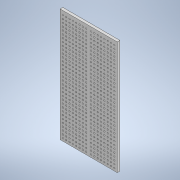
# Autodesk Inventor part: PCB_BOARD
Saved by Autodesk Inventor 2020 (Build 240168000, 168)
## iProperties
Created: 2020-06-08
Part Number: PCB_BOARD
Material: Generic
Document SubType Name: Modeling
Designer: Gebruiker
Density: 1 g/cm^3
Appearance: Default
Author: Gebruiker
Autodesk Inventor part; units mm, degrees
(part 1 of 2)
ref_plane "YZ Plane" through (0, 0, 0) normal (1, 0, 0) x (0, 1, 0)
ref_plane "XZ Plane" through (0, 0, 0) normal (0, 1, 0) x (-1, 0, 0)
ref_plane "XY Plane" through (0, 0, 0) normal (0, 0, 1) x (1, 0, 0)
sketch "Sketch1" plane through (0, 0, 0) normal (0, 0, 1) x (1, 0, 0)
  line L0 (-21.5, 42.5) -> (21.5, 42.5)
  line L1 (21.5, 42.5) -> (21.5, -42.5)
  line L2 (21.5, -42.5) -> (-21.5, -42.5)
  line L3 (-21.5, -42.5) -> (-21.5, 42.5)
  line L4 (-21.5, 32) -> (21.5, 32) construction
  line L5 (-21.7358, 34.5) -> (21.2642, 34.5) construction
  line L6 (-21.5945, 37) -> (21.4055, 37) construction
  line L7 (-33.8203, 0) -> (28.8511, 0) construction
  line L8 (-20.9841, 29.5) -> (22.0159, 29.5) construction
  line L9 (-20.1778, 24.5) -> (22.8222, 24.5) construction
  line L10 (-20.9207, 17) -> (22.0793, 17) construction
  line L11 (-20.9858, 19.5) -> (22.0142, 19.5) construction
  line L12 (-20.8573, 22) -> (22.1427, 22) construction
  line L13 (-21.1161, 27) -> (21.8839, 27) construction
  circle A0 centre (-19.3202, 39.5) radius 0.5
  circle A1 centre (-16.8202, 39.5) radius 0.5
  circle A2 centre (-14.3202, 39.5258) radius 0.5
  circle A3 centre (-11.8202, 39.5258) radius 0.5
  circle A4 centre (-9.3202, 39.5259) radius 0.5
  circle A5 centre (-6.8202, 39.5259) radius 0.5
  circle A6 centre (-4.3202, 39.5261) radius 0.5
  circle A7 centre (-1.8202, 39.5261) radius 0.5
  line L14 (0, 43.3712) -> (0, -59.117)
  circle A8 centre (19.3202, 39.5) radius 0.5
  circle A9 centre (16.8202, 39.5) radius 0.5
  circle A10 centre (14.3202, 39.5258) radius 0.5
  circle A11 centre (11.8202, 39.5258) radius 0.5
  circle A12 centre (9.3202, 39.5259) radius 0.5
  circle A13 centre (6.8202, 39.5259) radius 0.5
  circle A14 centre (1.8202, 39.5261) radius 0.5
  circle A15 centre (4.3202, 39.5261) radius 0.5
  line L15 (-21.5, 38.2501) -> (21.5, 38.2501) construction
  circle A16 centre (-19.3202, 37.0001) radius 0.5
  circle A17 centre (-16.8202, 37.0001) radius 0.5
  circle A18 centre (-14.3202, 36.9744) radius 0.5
  circle A19 centre (-11.8202, 36.9744) radius 0.5
  circle A20 centre (-9.3202, 36.9742) radius 0.5
  circle A21 centre (-6.8202, 36.9742) radius 0.5
  circle A22 centre (-1.8202, 36.9741) radius 0.5
  circle A23 centre (-4.3202, 36.9741) radius 0.5
  line L16 (0, 33.1289) -> (0, 135.6171)
  circle A24 centre (1.8202, 36.9741) radius 0.5
  circle A25 centre (4.3202, 36.9741) radius 0.5
  circle A26 centre (6.8202, 36.9742) radius 0.5
  circle A27 centre (9.3202, 36.9742) radius 0.5
  circle A28 centre (11.8202, 36.9744) radius 0.5
  circle A29 centre (14.3202, 36.9744) radius 0.5
  circle A30 centre (16.8202, 37.0001) radius 0.5
  circle A31 centre (19.3202, 37.0001) radius 0.5
  line L17 (-21.5945, 37) -> (0, 34.5) construction
  line L18 (0, 37) -> (-21.5, 34.5) construction
  line L19 (-21.5, 35.75) -> (21.5, 35.75) construction
  line L20 (-21.5945, 34.5) -> (21.4055, 34.5) construction
  circle A32 centre (-19.3202, 32) radius 0.5
  circle A33 centre (-16.8202, 32) radius 0.5
  circle A34 centre (-14.3202, 31.9742) radius 0.5
  circle A35 centre (-11.8202, 31.9742) radius 0.5
  circle A36 centre (-9.3202, 31.9741) radius 0.5
  circle A37 centre (-6.8202, 31.9741) radius 0.5
  circle A38 centre (-1.8202, 31.9739) radius 0.5
  circle A39 centre (-4.3202, 31.9739) radius 0.5
  line L21 (0, 28.1288) -> (0, 130.617)
  circle A40 centre (1.8202, 31.9739) radius 0.5
  circle A41 centre (4.3202, 31.9739) radius 0.5
  circle A42 centre (6.8202, 31.9741) radius 0.5
  circle A43 centre (9.3202, 31.9741) radius 0.5
  circle A44 centre (11.8202, 31.9742) radius 0.5
  circle A45 centre (14.3202, 31.9742) radius 0.5
  circle A46 centre (16.8202, 32) radius 0.5
  circle A47 centre (19.3202, 32) radius 0.5
  line L22 (-21.5, 33.2499) -> (21.5, 33.2499) construction
  circle A48 centre (1.8202, 34.5259) radius 0.5
  circle A49 centre (4.3202, 34.5259) radius 0.5
  circle A50 centre (6.8202, 34.5258) radius 0.5
  circle A51 centre (-1.8202, 34.5259) radius 0.5
  circle A52 centre (-4.3202, 34.5259) radius 0.5
  circle A53 centre (-9.3202, 34.5258) radius 0.5
  circle A54 centre (-6.8202, 34.5258) radius 0.5
  circle A55 centre (-11.8202, 34.5256) radius 0.5
  circle A56 centre (-14.3202, 34.5256) radius 0.5
  circle A57 centre (-16.8202, 34.4999) radius 0.5
  circle A58 centre (-19.3202, 34.4999) radius 0.5
  line L23 (0, 38.3711) -> (0, -64.1171)
  circle A59 centre (11.8202, 34.5256) radius 0.5
  circle A60 centre (14.3202, 34.5256) radius 0.5
  circle A61 centre (16.8202, 34.4999) radius 0.5
  circle A62 centre (19.3202, 34.4999) radius 0.5
  circle A63 centre (9.3202, 34.5258) radius 0.5
  line L24 (-21.5945, 34.5) -> (0, 37) construction
  line L25 (0, 34.5) -> (-21.5, 37) construction
  line L26 (-21.5, 32) -> (0, 29.5) construction
  line L27 (-21.5, 29.5) -> (0, 32) construction
  line L28 (-21.5, 30.75) -> (21.5, 30.75) construction
  line L29 (-21.5, 29.5) -> (21.5, 29.5) construction
  line L30 (-21.7358, 27) -> (21.2642, 27) construction
  line L31 (-21.5945, 24.5) -> (21.4055, 24.5) construction
  circle A64 centre (-19.3202, 22) radius 0.5
  circle A65 centre (-16.8202, 22) radius 0.5
  circle A66 centre (-14.3202, 21.9742) radius 0.5
  circle A67 centre (-11.8202, 21.9742) radius 0.5
  circle A68 centre (-9.3202, 21.9741) radius 0.5
  circle A69 centre (-6.8202, 21.9741) radius 0.5
  circle A70 centre (-1.8202, 21.9739) radius 0.5
  circle A71 centre (-4.3202, 21.9739) radius 0.5
  line L32 (0, 18.1288) -> (0, 120.617)
  circle A72 centre (1.8202, 21.9739) radius 0.5
  circle A73 centre (4.3202, 21.9739) radius 0.5
  circle A74 centre (6.8202, 21.9741) radius 0.5
  circle A75 centre (9.3202, 21.9741) radius 0.5
  circle A76 centre (11.8202, 21.9742) radius 0.5
  circle A77 centre (14.3202, 21.9742) radius 0.5
  circle A78 centre (16.8202, 22) radius 0.5
  circle A79 centre (19.3202, 22) radius 0.5
  line L33 (-21.5, 23.2499) -> (21.5, 23.2499) construction
  circle A80 centre (1.8202, 24.5259) radius 0.5
  circle A81 centre (4.3202, 24.5259) radius 0.5
  circle A82 centre (6.8202, 24.5258) radius 0.5
  circle A83 centre (-1.8202, 24.5259) radius 0.5
  circle A84 centre (-4.3202, 24.5259) radius 0.5
  circle A85 centre (-9.3202, 24.5258) radius 0.5
  circle A86 centre (-6.8202, 24.5258) radius 0.5
  circle A87 centre (-11.8202, 24.5256) radius 0.5
  circle A88 centre (-14.3202, 24.5256) radius 0.5
  circle A89 centre (-16.8202, 24.4999) radius 0.5
  circle A90 centre (-19.3202, 24.4999) radius 0.5
  line L34 (0, 28.3711) -> (0, -74.1171)
  circle A91 centre (11.8202, 24.5256) radius 0.5
  circle A92 centre (14.3202, 24.5256) radius 0.5
  circle A93 centre (16.8202, 24.4999) radius 0.5
  circle A94 centre (19.3202, 24.4999) radius 0.5
  circle A95 centre (9.3202, 24.5258) radius 0.5
  line L35 (-21.5945, 24.5) -> (0, 27) construction
  line L36 (0, 24.5) -> (-21.5, 27) construction
  line L37 (-21.5, 25.75) -> (21.5, 25.75) construction
  line L38 (0, 23.1289) -> (0, 125.6171)
  circle A96 centre (9.3202, 29.5259) radius 0.5
  line L39 (0, 33.3712) -> (0, -69.117)
  circle A97 centre (-19.3202, 29.5) radius 0.5
  circle A98 centre (-9.3202, 29.5259) radius 0.5
  circle A99 centre (-9.3202, 26.9742) radius 0.5
  circle A100 centre (-6.8202, 29.5259) radius 0.5
  circle A101 centre (-6.8202, 26.9742) radius 0.5
  circle A102 centre (-4.3202, 29.5261) radius 0.5
  circle A103 centre (-1.8202, 29.5261) radius 0.5
  circle A104 centre (-4.3202, 26.9741) radius 0.5
  circle A105 centre (-1.8202, 26.9741) radius 0.5
  circle A106 centre (1.8202, 26.9741) radius 0.5
  line L40 (-21.5945, 27) -> (0, 24.5) construction
  line L41 (0, 27) -> (-21.5, 24.5) construction
  line L42 (-21.5, 28.2501) -> (21.5, 28.2501) construction
  line L43 (-21.5945, 27) -> (21.4055, 27) construction
  circle A107 centre (4.3202, 29.5261) radius 0.5
  circle A108 centre (1.8202, 29.5261) radius 0.5
  circle A109 centre (6.8202, 29.5259) radius 0.5
  circle A110 centre (-14.3202, 26.9744) radius 0.5
  circle A111 centre (-14.3202, 29.5258) radius 0.5
  circle A112 centre (-16.8202, 29.5) radius 0.5
  circle A113 centre (-11.8202, 29.5258) radius 0.5
  circle A114 centre (14.3202, 29.5258) radius 0.5
  circle A115 centre (16.8202, 29.5) radius 0.5
  circle A116 centre (19.3202, 29.5) radius 0.5
  circle A117 centre (11.8202, 29.5258) radius 0.5
  circle A118 centre (-11.8202, 26.9744) radius 0.5
  circle A119 centre (6.8202, 26.9742) radius 0.5
  circle A120 centre (9.3202, 26.9742) radius 0.5
  circle A121 centre (4.3202, 26.9741) radius 0.5
  circle A122 centre (-19.3202, 27.0001) radius 0.5
  circle A123 centre (11.8202, 26.9744) radius 0.5
  circle A124 centre (14.3202, 26.9744) radius 0.5
  circle A125 centre (16.8202, 27.0001) radius 0.5
  circle A126 centre (19.3202, 27.0001) radius 0.5
  circle A127 centre (-16.8202, 27.0001) radius 0.5
  line L44 (-21.5, 29.5) -> (0, 32) construction
  line L45 (-21.5, 32) -> (0, 29.5) construction
  line L46 (-21.5, 22) -> (0, 19.5) construction
  line L47 (0, 22) -> (-21.5, 19.5) construction
  line L48 (-21.5, 20.75) -> (21.5, 20.75) construction
  line L49 (-20.8573, 19.5) -> (22.1427, 19.5) construction
  line L50 (0, -1.8712) -> (0, 100.617)
  line L51 (0, 3.1289) -> (0, 105.6171)
  circle A128 centre (-6.8202, 19.5259) radius 0.5
  circle A129 centre (-11.8202, 19.5258) radius 0.5
  circle A130 centre (-14.3202, 19.5258) radius 0.5
  circle A131 centre (-9.3202, 19.5259) radius 0.5
  circle A132 centre (-19.3202, 19.5) radius 0.5
  circle A133 centre (-16.8202, 19.5) radius 0.5
  line L52 (0, 23.3712) -> (0, -79.117)
  circle A134 centre (-4.3202, 19.5261) radius 0.5
  circle A135 centre (-1.8202, 19.5261) radius 0.5
  circle A136 centre (9.3202, 19.5259) radius 0.5
  line L53 (0, 13.1289) -> (0, 115.6171)
  line L54 (0, 8.1288) -> (0, 110.617)
  circle A137 centre (1.8202, 19.5261) radius 0.5
  circle A138 centre (4.3202, 19.5261) radius 0.5
  circle A139 centre (6.8202, 19.5259) radius 0.5
  circle A140 centre (11.8202, 19.5258) radius 0.5
  circle A141 centre (14.3202, 19.5258) radius 0.5
  circle A142 centre (16.8202, 19.5) radius 0.5
  circle A143 centre (19.3202, 19.5) radius 0.5
  line L55 (-21.5, 19.5) -> (0, 22) construction
  line L56 (0, 19.5) -> (-21.5, 22) construction
  line L57 (-21.5, 19.5) -> (0, 17) construction
  line L58 (0, 19.5) -> (-21.5, 17) construction
  line L59 (-21.5, 17) -> (-21.5, 18.25) construction
  line L60 (-21.5, 18.25) -> (21.5, 18.25) construction
  line L61 (-21.5, 4.5) -> (21.5, 4.5) construction
  line L62 (-21.7358, 2) -> (21.2642, 2) construction
  line L63 (-21.5945, -0.5) -> (21.4055, -0.5) construction
  line L64 (-20.9841, 7) -> (22.0159, 7) construction
  line L65 (-20.1778, 12) -> (22.8222, 12) construction
  line L66 (-20.9858, 17) -> (22.0142, 17) construction
  line L67 (-20.8573, 14.5) -> (22.1427, 14.5) construction
  line L68 (-21.1161, 9.5) -> (21.8839, 9.5) construction
  circle A144 centre (-19.3202, -3) radius 0.5
  circle A145 centre (-16.8202, -3) radius 0.5
  circle A146 centre (-14.3202, -3.0258) radius 0.5
  circle A147 centre (-11.8202, -3.0258) radius 0.5
  circle A148 centre (-9.3202, -3.0259) radius 0.5
  circle A149 centre (-6.8202, -3.0259) radius 0.5
  circle A150 centre (-1.8202, -3.0261) radius 0.5
  circle A151 centre (-4.3202, -3.0261) radius 0.5
  line L69 (0, -6.8712) -> (0, 95.617)
  circle A152 centre (1.8202, -3.0261) radius 0.5
  circle A153 centre (4.3202, -3.0261) radius 0.5
  circle A154 centre (6.8202, -3.0259) radius 0.5
  circle A155 centre (9.3202, -3.0259) radius 0.5
  circle A156 centre (11.8202, -3.0258) radius 0.5
  circle A157 centre (14.3202, -3.0258) radius 0.5
  circle A158 centre (16.8202, -3) radius 0.5
  circle A159 centre (19.3202, -3) radius 0.5
  line L70 (-21.5, -1.7501) -> (21.5, -1.7501) construction
  circle A160 centre (1.8202, -0.4741) radius 0.5
  circle A161 centre (4.3202, -0.4741) radius 0.5
  circle A162 centre (6.8202, -0.4742) radius 0.5
  circle A163 centre (-1.8202, -0.4741) radius 0.5
  circle A164 centre (-4.3202, -0.4741) radius 0.5
  circle A165 centre (-9.3202, -0.4742) radius 0.5
  circle A166 centre (-6.8202, -0.4742) radius 0.5
  circle A167 centre (-11.8202, -0.4744) radius 0.5
  circle A168 centre (-14.3202, -0.4744) radius 0.5
  circle A169 centre (-16.8202, -0.5001) radius 0.5
  circle A170 centre (-19.3202, -0.5001) radius 0.5
  line L71 (0, 3.3711) -> (0, -99.1171)
  circle A171 centre (11.8202, -0.4744) radius 0.5
  circle A172 centre (14.3202, -0.4744) radius 0.5
  circle A173 centre (16.8202, -0.5001) radius 0.5
  circle A174 centre (19.3202, -0.5001) radius 0.5
  circle A175 centre (9.3202, -0.4742) radius 0.5
  line L72 (-21.5945, -0.5) -> (0, 2) construction
  line L73 (0, -0.5) -> (-21.5, 2) construction
  line L74 (-21.5, 0.75) -> (21.5, 0.75) construction
  line L75 (0, -1.8711) -> (0, 100.6171)
  circle A176 centre (9.3202, 4.5259) radius 0.5
  line L76 (0, 8.3712) -> (0, -94.117)
  circle A177 centre (-19.3202, 4.5) radius 0.5
  circle A178 centre (-9.3202, 4.5259) radius 0.5
  circle A179 centre (-9.3202, 1.9742) radius 0.5
  circle A180 centre (-6.8202, 4.5259) radius 0.5
  circle A181 centre (-6.8202, 1.9742) radius 0.5
  circle A182 centre (-4.3202, 4.5261) radius 0.5
  circle A183 centre (-1.8202, 4.5261) radius 0.5
  circle A184 centre (-4.3202, 1.9741) radius 0.5
  circle A185 centre (-1.8202, 1.9741) radius 0.5
  circle A186 centre (1.8202, 1.9741) radius 0.5
  line L77 (-21.5945, 2) -> (0, -0.5) construction
  line L78 (0, 2) -> (-21.5, -0.5) construction
  line L79 (-21.5, 3.2501) -> (21.5, 3.2501) construction
  line L80 (-21.5945, 2) -> (21.4055, 2) construction
  circle A187 centre (4.3202, 4.5261) radius 0.5
  circle A188 centre (1.8202, 4.5261) radius 0.5
  circle A189 centre (6.8202, 4.5259) radius 0.5
  circle A190 centre (-14.3202, 1.9744) radius 0.5
  circle A191 centre (-14.3202, 4.5258) radius 0.5
  circle A192 centre (-16.8202, 4.5) radius 0.5
  circle A193 centre (-11.8202, 4.5258) radius 0.5
  circle A194 centre (14.3202, 4.5258) radius 0.5
  circle A195 centre (16.8202, 4.5) radius 0.5
  circle A196 centre (19.3202, 4.5) radius 0.5
  circle A197 centre (11.8202, 4.5258) radius 0.5
  circle A198 centre (-11.8202, 1.9744) radius 0.5
  circle A199 centre (6.8202, 1.9742) radius 0.5
  circle A200 centre (9.3202, 1.9742) radius 0.5
  circle A201 centre (4.3202, 1.9741) radius 0.5
  circle A202 centre (-19.3202, 2.0001) radius 0.5
  circle A203 centre (11.8202, 1.9744) radius 0.5
  circle A204 centre (14.3202, 1.9744) radius 0.5
  circle A205 centre (16.8202, 2.0001) radius 0.5
  circle A206 centre (19.3202, 2.0001) radius 0.5
  circle A207 centre (-16.8202, 2.0001) radius 0.5
  line L81 (-21.5, 4.5) -> (0, 7) construction
  line L82 (-21.5, 7) -> (0, 4.5) construction
  line L83 (-21.5, 5.75) -> (21.5, 5.75) construction
  circle A208 centre (-6.8202, 11.9742) radius 0.5
  circle A209 centre (-6.8202, 14.5259) radius 0.5
  circle A210 centre (-11.8202, 6.9742) radius 0.5
  circle A211 centre (-11.8202, 11.9744) radius 0.5
  circle A212 centre (-11.8202, 14.5258) radius 0.5
  circle A213 centre (-14.3202, 14.5258) radius 0.5
  circle A214 centre (-11.8202, 9.5256) radius 0.5
  circle A215 centre (-14.3202, 6.9742) radius 0.5
  circle A216 centre (-9.3202, 9.5258) radius 0.5
  circle A217 centre (-9.3202, 6.9741) radius 0.5
  circle A218 centre (-6.8202, 9.5258) radius 0.5
  circle A219 centre (-6.8202, 6.9741) radius 0.5
  circle A220 centre (-4.3202, 9.5259) radius 0.5
  circle A221 centre (-4.3202, 6.9739) radius 0.5
  line L84 (0, 12) -> (-21.5, 9.5) construction
  line L85 (0, 9.5) -> (-21.5, 12) construction
  line L86 (-21.5945, 12) -> (0, 9.5) construction
  line L87 (-21.5945, 9.5) -> (0, 12) construction
  line L88 (-21.5, 7) -> (0, 4.5) construction
  line L89 (-21.5, 4.5) -> (0, 7) construction
  circle A222 centre (-9.3202, 14.5259) radius 0.5
  circle A223 centre (-9.3202, 11.9742) radius 0.5
  circle A224 centre (-16.8202, 7) radius 0.5
  circle A225 centre (-19.3202, 7) radius 0.5
  circle A226 centre (-19.3202, 14.5) radius 0.5
  circle A227 centre (-19.3202, 9.4999) radius 0.5
  circle A228 centre (-19.3202, 12.0001) radius 0.5
  circle A229 centre (-16.8202, 14.5) radius 0.5
  circle A230 centre (-16.8202, 12.0001) radius 0.5
  line L90 (-21.5945, 12) -> (21.4055, 12) construction
  line L91 (-21.7358, 9.5) -> (21.2642, 9.5) construction
  line L92 (-21.5, 13.2501) -> (21.5, 13.2501) construction
  circle A231 centre (-14.3202, 11.9744) radius 0.5
  circle A232 centre (-1.8202, 11.9741) radius 0.5
  circle A233 centre (-4.3202, 11.9741) radius 0.5
  circle A234 centre (4.3202, 11.9741) radius 0.5
  line L93 (0, 13.3711) -> (0, -89.1171)
  line L94 (0, 18.3712) -> (0, -84.117)
  line L95 (-21.5, 7) -> (21.5, 7) construction
  circle A235 centre (1.8202, 11.9741) radius 0.5
  circle A236 centre (-4.3202, 14.5261) radius 0.5
  circle A237 centre (-1.8202, 14.5261) radius 0.5
  circle A238 centre (-1.8202, 6.9739) radius 0.5
  circle A239 centre (-1.8202, 9.5259) radius 0.5
  circle A240 centre (1.8202, 9.5259) radius 0.5
  circle A241 centre (4.3202, 6.9739) radius 0.5
  circle A242 centre (4.3202, 9.5259) radius 0.5
  circle A243 centre (1.8202, 6.9739) radius 0.5
  circle A244 centre (6.8202, 11.9742) radius 0.5
  line L96 (-21.5945, 9.5) -> (21.4055, 9.5) construction
  line L97 (-21.5, 10.75) -> (21.5, 10.75) construction
  line L98 (-21.5, 8.2499) -> (21.5, 8.2499) construction
  circle A245 centre (-14.3202, 9.5256) radius 0.5
  circle A246 centre (9.3202, 14.5259) radius 0.5
  line L99 (0, 8.1289) -> (0, 110.6171)
  line L100 (0, 3.1288) -> (0, 105.617)
  circle A247 centre (-16.8202, 9.4999) radius 0.5
  circle A248 centre (1.8202, 14.5261) radius 0.5
  circle A249 centre (4.3202, 14.5261) radius 0.5
  circle A250 centre (6.8202, 14.5259) radius 0.5
  circle A251 centre (11.8202, 14.5258) radius 0.5
  circle A252 centre (14.3202, 14.5258) radius 0.5
  circle A253 centre (16.8202, 14.5) radius 0.5
  circle A254 centre (19.3202, 14.5) radius 0.5
  circle A255 centre (16.8202, 12.0001) radius 0.5
  circle A256 centre (14.3202, 11.9744) radius 0.5
  circle A257 centre (19.3202, 12.0001) radius 0.5
  circle A258 centre (11.8202, 11.9744) radius 0.5
  circle A259 centre (9.3202, 11.9742) radius 0.5
  circle A260 centre (6.8202, 6.9741) radius 0.5
  circle A261 centre (14.3202, 6.9742) radius 0.5
  circle A262 centre (6.8202, 9.5258) radius 0.5
  circle A263 centre (9.3202, 9.5258) radius 0.5
  circle A264 centre (11.8202, 9.5256) radius 0.5
  circle A265 centre (11.8202, 6.9742) radius 0.5
  circle A266 centre (14.3202, 9.5256) radius 0.5
  circle A267 centre (16.8202, 7) radius 0.5
  circle A268 centre (16.8202, 9.4999) radius 0.5
  circle A269 centre (19.3202, 9.4999) radius 0.5
  circle A270 centre (19.3202, 7) radius 0.5
  circle A271 centre (9.3202, 6.9741) radius 0.5
  line L101 (-21.5, 14.5) -> (0, 17) construction
  line L102 (0, 14.5) -> (-21.5, 17) construction
  line L103 (-21.5, 15.75) -> (21.5, 15.75) construction
  line L104 (0, 13.1288) -> (0, 115.617)
  line L105 (-20.8573, 17) -> (22.1427, 17) construction
  circle A272 centre (-19.3202, 17) radius 0.5
  circle A273 centre (-4.3202, 16.9739) radius 0.5
  line L106 (0, 38.3712) -> (0, -64.117)
  line L107 (0, 33.3711) -> (0, -69.1171)
  line L108 (0, 28.3712) -> (0, -74.117)
  line L109 (0, 23.3711) -> (0, -79.1171)
  circle A274 centre (-6.8202, 16.9741) radius 0.5
  circle A275 centre (-1.8202, 16.9739) radius 0.5
  circle A276 centre (-9.3202, 16.9741) radius 0.5
  circle A277 centre (-11.8202, 16.9742) radius 0.5
  circle A278 centre (-14.3202, 16.9742) radius 0.5
  line L110 (0, 17) -> (-21.5, 14.5) construction
  line L111 (-21.5, 17) -> (0, 14.5) construction
  circle A279 centre (-16.8202, 17) radius 0.5
  circle A280 centre (4.3202, 16.9739) radius 0.5
  circle A281 centre (6.8202, 16.9741) radius 0.5
  circle A282 centre (9.3202, 16.9741) radius 0.5
  circle A283 centre (11.8202, 16.9742) radius 0.5
  circle A284 centre (1.8202, 16.9739) radius 0.5
  circle A285 centre (14.3202, 16.9742) radius 0.5
  circle A286 centre (16.8202, 17) radius 0.5
  circle A287 centre (19.3202, 17) radius 0.5
  line L112 (-21.5, 17) -> (0, 19.5) construction
  line L113 (0, 17) -> (-21.5, 19.5) construction
  line L114 (-33.8203, -3.5001) -> (28.8511, -3.5001) construction
  line L115 (-20.9207, -20.5001) -> (22.0793, -20.5001) construction
  line L116 (0, -46.8713) -> (0, 55.6168)
  line L117 (0, -41.8712) -> (0, 60.617)
  line L118 (0, -31.8712) -> (0, 70.617)
  line L119 (0, -36.8713) -> (0, 65.6168)
  line L120 (0, -26.8713) -> (0, 75.6168)
  line L121 (0, -1.6289) -> (0, -104.1171)
  line L122 (0, -6.6291) -> (0, -109.1173)
  line L123 (0, -11.6289) -> (0, -114.1171)
  line L124 (0, -16.6291) -> (0, -119.1173)
  line L125 (-21.5, -23.0001) -> (0, -20.5001) construction
  line L126 (0, -23.0001) -> (-21.5, -20.5001) construction
  circle A288 centre (4.3202, -13.0261) radius 0.5
  circle A289 centre (4.3202, -10.4741) radius 0.5
  circle A290 centre (1.8202, -5.4742) radius 0.5
  circle A291 centre (4.3202, -3.0261) radius 0.5
  circle A292 centre (9.3202, -3.0259) radius 0.5
  circle A293 centre (14.3202, -3.0258) radius 0.5
  circle A294 centre (11.8202, -3.0258) radius 0.5
  circle A295 centre (16.8202, -3) radius 0.5
  circle A296 centre (-1.8202, -5.4742) radius 0.5
  circle A297 centre (-1.8202, -3.0261) radius 0.5
  circle A298 centre (-4.3202, -3.0261) radius 0.5
  line L127 (-21.5, -19.2501) -> (21.5, -19.2501) construction
  line L128 (-21.5, -14.2501) -> (21.5, -14.2501) construction
  line L129 (-21.5945, -5.5001) -> (21.4055, -5.5001) construction
  circle A299 centre (-9.3202, -3.0259) radius 0.5
  circle A300 centre (-11.8202, -3.0258) radius 0.5
  circle A301 centre (-14.3202, -3.0258) radius 0.5
  circle A302 centre (-16.8202, -3) radius 0.5
  circle A303 centre (-6.8202, -3.0259) radius 0.5
  line L130 (-20.1778, -15.5001) -> (22.8222, -15.5001) construction
  line L131 (-20.8573, -18.0001) -> (22.1427, -18.0001) construction
  line L132 (-20.8573, -20.5001) -> (22.1427, -20.5001) construction
  line L133 (-20.9841, -10.5001) -> (22.0159, -10.5001) construction
  line L134 (-20.9858, -20.5001) -> (22.0142, -20.5001) construction
  line L135 (-21.1161, -13.0001) -> (21.8839, -13.0001) construction
  line L136 (-21.5, -11.7501) -> (21.5, -11.7501) construction
  line L137 (-21.5, -8.0001) -> (21.5, -8.0001) construction
  line L138 (-21.5945, -3.0001) -> (21.4055, -3.0001) construction
  line L139 (-21.7358, -5.5001) -> (21.2642, -5.5001) construction
  circle A304 centre (1.8202, -3.0261) radius 0.5
  circle A305 centre (6.8202, -3.0259) radius 0.5
  line L140 (0, -41.8713) -> (0, 60.6168)
  line L141 (0, -6.8712) -> (0, 95.617)
  line L142 (0, -36.8712) -> (0, 65.617)
  line L143 (0, -31.8713) -> (0, 70.6168)
  line L144 (0, -26.8712) -> (0, 75.617)
  line L145 (0, -21.8713) -> (0, 80.6168)
  line L146 (0, -16.8712) -> (0, 85.617)
  line L147 (0, -11.8713) -> (0, 90.6168)
  circle A306 centre (-16.8202, -8.0001) radius 0.5
  circle A307 centre (-19.3202, -3) radius 0.5
  circle A308 centre (19.3202, -3) radius 0.5
  circle A309 centre (-4.3202, -5.4742) radius 0.5
  circle A310 centre (9.3202, -18.0261) radius 0.5
  circle A311 centre (-14.3202, -18.0259) radius 0.5
  circle A312 centre (-6.8202, -5.4744) radius 0.5
  circle A313 centre (-6.8202, -8.0261) radius 0.5
  circle A314 centre (-9.3202, -5.4744) radius 0.5
  circle A315 centre (-9.3202, -8.0261) radius 0.5
  line L148 (0, -3.0001) -> (-21.5, -5.5001) construction
  line L149 (0, -5.5001) -> (-21.5, -3.0001) construction
  line L150 (-21.5945, -3.0001) -> (0, -5.5001) construction
  line L151 (-21.5945, -5.5001) -> (0, -3.0001) construction
  circle A316 centre (-19.3202, -8.0001) radius 0.5
  line L152 (-21.5, -4.2501) -> (21.5, -4.2501) construction
  circle A317 centre (-19.3202, -5.5003) radius 0.5
  circle A318 centre (-16.8202, -5.5003) radius 0.5
  circle A319 centre (-14.3202, -5.4745) radius 0.5
  circle A320 centre (-11.8202, -5.4745) radius 0.5
  circle A321 centre (-4.3202, -8.0262) radius 0.5
  circle A322 centre (-1.8202, -8.0262) radius 0.5
  circle A323 centre (4.3202, -5.4742) radius 0.5
  circle A324 centre (6.8202, -5.4744) radius 0.5
  circle A325 centre (9.3202, -8.0261) radius 0.5
  circle A326 centre (9.3202, -5.4744) radius 0.5
  circle A327 centre (11.8202, -5.4745) radius 0.5
  circle A328 centre (14.3202, -5.4745) radius 0.5
  circle A329 centre (1.8202, -10.4741) radius 0.5
  circle A330 centre (16.8202, -5.5003) radius 0.5
  circle A331 centre (19.3202, -5.5003) radius 0.5
  circle A332 centre (6.8202, -10.4742) radius 0.5
  circle A333 centre (-1.8202, -13.0261) radius 0.5
  circle A334 centre (1.8202, -13.0261) radius 0.5
  circle A335 centre (-4.3202, -18.0262) radius 0.5
  circle A336 centre (-1.8202, -18.0262) radius 0.5
  circle A337 centre (1.8202, -20.4741) radius 0.5
  circle A338 centre (19.3202, -15.5003) radius 0.5
  circle A339 centre (-11.8202, -15.4745) radius 0.5
  circle A340 centre (-6.8202, -15.4744) radius 0.5
  circle A341 centre (-6.8202, -18.0261) radius 0.5
  circle A342 centre (-4.3202, -10.4741) radius 0.5
  circle A343 centre (6.8202, -20.4742) radius 0.5
  circle A344 centre (9.3202, -15.4744) radius 0.5
  circle A345 centre (6.8202, -13.0259) radius 0.5
  circle A346 centre (6.8202, -18.0261) radius 0.5
  circle A347 centre (4.3202, -15.4742) radius 0.5
  circle A348 centre (4.3202, -18.0262) radius 0.5
  circle A349 centre (1.8202, -18.0262) radius 0.5
  circle A350 centre (9.3202, -13.0259) radius 0.5
  circle A351 centre (11.8202, -8.0259) radius 0.5
  circle A352 centre (16.8202, -8.0001) radius 0.5
  line L153 (-21.5945, -15.5001) -> (0, -13.0001) construction
  line L154 (-21.5945, -13.0001) -> (0, -15.5001) construction
  line L155 (-21.5945, -15.5001) -> (21.4055, -15.5001) construction
  line L156 (-21.7358, -13.0001) -> (21.2642, -13.0001) construction
  line L157 (-21.5945, -13.0001) -> (21.4055, -13.0001) construction
  circle A353 centre (14.3202, -8.0259) radius 0.5
  circle A354 centre (19.3202, -8.0001) radius 0.5
  line L158 (-21.5, -10.5001) -> (21.5, -10.5001) construction
  line L159 (-21.5, -6.7502) -> (21.5, -6.7502) construction
  line L160 (-21.5, -20.5001) -> (0, -23.0001) construction
  line L161 (-21.5, -16.7502) -> (21.5, -16.7502) construction
  line L162 (-21.5, -9.2501) -> (21.5, -9.2501) construction
  circle A355 centre (-4.3202, -13.0261) radius 0.5
  circle A356 centre (-9.3202, -13.0259) radius 0.5
  circle A357 centre (-6.8202, -13.0259) radius 0.5
  line L163 (-21.5, -10.5001) -> (0, -8.0001) construction
  line L164 (-21.5, -8.0001) -> (0, -10.5001) construction
  circle A358 centre (6.8202, -8.0261) radius 0.5
  circle A359 centre (4.3202, -8.0262) radius 0.5
  circle A360 centre (1.8202, -8.0262) radius 0.5
  circle A361 centre (-14.3202, -8.0259) radius 0.5
  circle A362 centre (-11.8202, -8.0259) radius 0.5
  circle A363 centre (-11.8202, -18.0259) radius 0.5
  line L165 (0, 3.3711) -> (0, -99.1171)
  line L166 (0, -1.6291) -> (0, -104.1173)
  line L167 (0, -6.6289) -> (0, -109.1171)
  line L168 (0, -11.6291) -> (0, -114.1173)
  line L169 (0, -16.6289) -> (0, -119.1171)
  circle A364 centre (9.3202, -20.4742) radius 0.5
  circle A365 centre (11.8202, -20.4744) radius 0.5
  circle A366 centre (14.3202, -20.4744) radius 0.5
  circle A367 centre (16.8202, -20.5001) radius 0.5
  circle A368 centre (19.3202, -20.5001) radius 0.5
  circle A369 centre (4.3202, -20.4741) radius 0.5
  circle A370 centre (-16.8202, -10.5001) radius 0.5
  circle A371 centre (-11.8202, -10.4744) radius 0.5
  circle A372 centre (-11.8202, -13.0258) radius 0.5
  circle A373 centre (-9.3202, -10.4742) radius 0.5
  circle A374 centre (-6.8202, -10.4742) radius 0.5
  circle A375 centre (6.8202, -15.4744) radius 0.5
  circle A376 centre (11.8202, -10.4744) radius 0.5
  circle A377 centre (14.3202, -10.4744) radius 0.5
  circle A378 centre (11.8202, -18.0259) radius 0.5
  circle A379 centre (11.8202, -15.4745) radius 0.5
  circle A380 centre (11.8202, -13.0258) radius 0.5
  circle A381 centre (14.3202, -18.0259) radius 0.5
  circle A382 centre (14.3202, -13.0258) radius 0.5
  circle A383 centre (14.3202, -15.4745) radius 0.5
  circle A384 centre (19.3202, -18.0001) radius 0.5
  circle A385 centre (9.3202, -10.4742) radius 0.5
  circle A386 centre (19.3202, -13) radius 0.5
  circle A387 centre (19.3202, -10.5001) radius 0.5
  circle A388 centre (-19.3202, -10.5001) radius 0.5
  circle A389 centre (-1.8202, -10.4741) radius 0.5
  circle A390 centre (-1.8202, -20.4741) radius 0.5
  circle A391 centre (-14.3202, -10.4744) radius 0.5
  line L170 (0, -18.0001) -> (-21.5, -20.5001) construction
  line L171 (-21.5, -20.5001) -> (0, -18.0001) construction
  line L172 (-21.5, -8.0001) -> (0, -10.5001) construction
  line L173 (-21.5, -10.5001) -> (0, -8.0001) construction
  circle A392 centre (-19.3202, -13) radius 0.5
  circle A393 centre (-14.3202, -13.0258) radius 0.5
  circle A394 centre (-14.3202, -15.4745) radius 0.5
  circle A395 centre (-16.8202, -20.5001) radius 0.5
  circle A396 centre (-16.8202, -18.0001) radius 0.5
  circle A397 centre (-16.8202, -15.5003) radius 0.5
  circle A398 centre (-16.8202, -13) radius 0.5
  circle A399 centre (-19.3202, -20.5001) radius 0.5
  circle A400 centre (-19.3202, -18.0001) radius 0.5
  circle A401 centre (-19.3202, -15.5003) radius 0.5
  circle A402 centre (-14.3202, -20.4744) radius 0.5
  circle A403 centre (-11.8202, -20.4744) radius 0.5
  line L174 (0, -15.5001) -> (-21.5, -13.0001) construction
  line L175 (0, -13.0001) -> (-21.5, -15.5001) construction
  line L176 (0, -20.5001) -> (-21.5, -18.0001) construction
  line L177 (-21.5, -18.0001) -> (0, -20.5001) construction
  line L178 (0, -20.5001) -> (-21.5, -23.0001) construction
  circle A404 centre (-9.3202, -20.4742) radius 0.5
  circle A405 centre (-9.3202, -18.0261) radius 0.5
  circle A406 centre (-9.3202, -15.4744) radius 0.5
  circle A407 centre (-6.8202, -20.4742) radius 0.5
  circle A408 centre (-4.3202, -20.4741) radius 0.5
  circle A409 centre (-4.3202, -15.4742) radius 0.5
  circle A410 centre (-1.8202, -15.4742) radius 0.5
  circle A411 centre (16.8202, -18.0001) radius 0.5
  circle A412 centre (16.8202, -15.5003) radius 0.5
  circle A413 centre (16.8202, -13) radius 0.5
  circle A414 centre (16.8202, -10.5001) radius 0.5
  circle A415 centre (1.8202, -15.4742) radius 0.5
  line L179 (0, -81.8715) -> (0, 20.6167)
  line L180 (0, -76.8713) -> (0, 25.6168)
  line L181 (0, -66.8713) -> (0, 35.6168)
  line L182 (0, -71.8715) -> (0, 30.6167)
  line L183 (0, -61.8715) -> (0, 40.6167)
  circle A416 centre (11.8202, -35.4745) radius 0.5
  circle A417 centre (9.3202, -35.4744) radius 0.5
  circle A418 centre (6.8202, -35.4744) radius 0.5
  circle A419 centre (-1.8202, -35.4742) radius 0.5
  circle A420 centre (-6.8202, -35.4744) radius 0.5
  circle A421 centre (-9.3202, -35.4744) radius 0.5
  circle A422 centre (-11.8202, -35.4745) radius 0.5
  circle A423 centre (-14.3202, -35.4745) radius 0.5
  circle A424 centre (-16.8202, -35.5003) radius 0.5
  circle A425 centre (-19.3202, -35.5003) radius 0.5
  circle A426 centre (-4.3202, -35.4742) radius 0.5
  circle A427 centre (1.8202, -35.4742) radius 0.5
  circle A428 centre (4.3202, -35.4742) radius 0.5
  circle A429 centre (14.3202, -35.4745) radius 0.5
  circle A430 centre (19.3202, -35.5003) radius 0.5
  line L184 (0, -76.8715) -> (0, 25.6167)
  line L185 (0, -41.8713) -> (0, 60.6168)
  line L186 (0, -71.8713) -> (0, 30.6168)
  line L187 (0, -66.8715) -> (0, 35.6167)
  line L188 (0, -61.8713) -> (0, 40.6168)
  line L189 (0, -56.8715) -> (0, 45.6167)
  line L190 (0, -51.8713) -> (0, 50.6168)
  line L191 (0, -46.8715) -> (0, 55.6167)
  circle A431 centre (16.8202, -35.5003) radius 0.5
  line L192 (0, -31.6291) -> (0, -134.1173)
  line L193 (0, -41.8713) -> (0, 60.6168)
  line L194 (0, -21.8712) -> (0, 80.617)
  line L195 (0, -21.8713) -> (0, 80.6168)
  line L196 (0, -26.8712) -> (0, 75.617)
  line L197 (0, -26.8713) -> (0, 75.6168)
  line L198 (0, -36.8713) -> (0, 65.6168)
  line L199 (0, -36.8712) -> (0, 65.617)
  line L200 (0, -31.8712) -> (0, 70.617)
  line L201 (0, -31.8713) -> (0, 70.6168)
  circle A432 centre (1.8202, -20.4741) radius 0.5
  circle A433 centre (4.3202, -23.0261) radius 0.5
  circle A434 centre (4.3202, -20.4741) radius 0.5
  circle A435 centre (1.8202, -28.0262) radius 0.5
  circle A436 centre (16.8202, -35.5003) radius 0.5
  circle A437 centre (19.3202, -35.5003) radius 0.5
  circle A438 centre (9.3202, -30.4742) radius 0.5
  circle A439 centre (9.3202, -33.0259) radius 0.5
  circle A440 centre (6.8202, -33.0259) radius 0.5
  circle A441 centre (11.8202, -33.0258) radius 0.5
  line L202 (-21.5, -28.0001) -> (21.5, -28.0001) construction
  circle A442 centre (9.3202, -20.4742) radius 0.5
  line L203 (-21.5, -21.7501) -> (21.5, -21.7501) construction
  line L204 (-20.8573, -20.5001) -> (22.1427, -20.5001) construction
  line L205 (-20.1778, -23.0001) -> (22.8222, -23.0001) construction
  line L206 (-20.9841, -28.0001) -> (22.0159, -28.0001) construction
  circle A443 centre (4.3202, -25.4742) radius 0.5
  circle A444 centre (-16.8202, -35.5003) radius 0.5
  circle A445 centre (4.3202, -28.0262) radius 0.5
  circle A446 centre (1.8202, -33.0261) radius 0.5
  circle A447 centre (-1.8202, -30.4741) radius 0.5
  circle A448 centre (-4.3202, -30.4741) radius 0.5
  circle A449 centre (4.3202, -33.0261) radius 0.5
  circle A450 centre (6.8202, -28.0261) radius 0.5
  circle A451 centre (-4.3202, -28.0262) radius 0.5
  line L207 (-21.7358, -33.0001) -> (21.2642, -33.0001) construction
  line L208 (-21.7358, -25.5001) -> (21.2642, -25.5001) construction
  line L209 (-21.5945, -35.5001) -> (21.4055, -35.5001) construction
  line L210 (-21.5945, -25.5001) -> (21.4055, -25.5001) construction
  line L211 (-33.8203, -35.0001) -> (28.8511, -35.0001) construction
  circle A452 centre (4.3202, -35.4742) radius 0.5
  circle A453 centre (9.3202, -35.4744) radius 0.5
  circle A454 centre (14.3202, -35.4745) radius 0.5
  line L212 (-21.5, -26.7502) -> (21.5, -26.7502) construction
  line L213 (-21.5, -29.2501) -> (21.5, -29.2501) construction
  line L214 (-21.5, -31.7501) -> (21.5, -31.7501) construction
  line L215 (-21.5, -34.2501) -> (21.5, -34.2501) construction
  circle A455 centre (1.8202, -35.4742) radius 0.5
  circle A456 centre (-9.3202, -35.4744) radius 0.5
  circle A457 centre (6.8202, -35.4744) radius 0.5
  circle A458 centre (11.8202, -35.4745) radius 0.5
  circle A459 centre (-11.8202, -35.4745) radius 0.5
  circle A460 centre (-14.3202, -35.4745) radius 0.5
  line L216 (-21.1161, -25.5001) -> (21.8839, -25.5001) construction
  line L217 (-21.5945, -33.0001) -> (21.4055, -33.0001) construction
  circle A461 centre (16.8202, -23) radius 0.5
  circle A462 centre (14.3202, -23.0258) radius 0.5
  circle A463 centre (16.8202, -25.5003) radius 0.5
  circle A464 centre (19.3202, -25.5003) radius 0.5
  circle A465 centre (19.3202, -28.0001) radius 0.5
  circle A466 centre (14.3202, -25.4745) radius 0.5
  circle A467 centre (16.8202, -28.0001) radius 0.5
  circle A468 centre (14.3202, -28.0259) radius 0.5
  circle A469 centre (14.3202, -33.0258) radius 0.5
  circle A470 centre (19.3202, -33) radius 0.5
  circle A471 centre (16.8202, -33) radius 0.5
  circle A472 centre (6.8202, -20.4742) radius 0.5
  circle A473 centre (6.8202, -25.4744) radius 0.5
  circle A474 centre (9.3202, -23.0259) radius 0.5
  circle A475 centre (9.3202, -25.4744) radius 0.5
  circle A476 centre (11.8202, -30.4744) radius 0.5
  circle A477 centre (-4.3202, -25.4742) radius 0.5
  circle A478 centre (6.8202, -23.0259) radius 0.5
  circle A479 centre (11.8202, -23.0258) radius 0.5
  circle A480 centre (11.8202, -25.4745) radius 0.5
  circle A481 centre (9.3202, -28.0261) radius 0.5
  circle A482 centre (1.8202, -23.0261) radius 0.5
  circle A483 centre (11.8202, -28.0259) radius 0.5
  circle A484 centre (-1.8202, -23.0261) radius 0.5
  circle A485 centre (-4.3202, -23.0261) radius 0.5
  circle A486 centre (16.8202, -30.5001) radius 0.5
  circle A487 centre (14.3202, -30.4744) radius 0.5
  circle A488 centre (19.3202, -30.5001) radius 0.5
  circle A489 centre (6.8202, -30.4742) radius 0.5
  circle A490 centre (4.3202, -30.4741) radius 0.5
  circle A491 centre (1.8202, -30.4741) radius 0.5
  circle A492 centre (16.8202, -20.5001) radius 0.5
  circle A493 centre (14.3202, -20.4744) radius 0.5
  circle A494 centre (11.8202, -20.4744) radius 0.5
  circle A495 centre (19.3202, -20.5001) radius 0.5
  circle A496 centre (1.8202, -25.4742) radius 0.5
  circle A497 centre (19.3202, -23) radius 0.5
  line L218 (-21.5, -24.2501) -> (21.5, -24.2501) construction
  line L219 (-21.5, -30.5001) -> (21.5, -30.5001) construction
  line L220 (-21.5945, -23.0001) -> (21.4055, -23.0001) construction
  circle A498 centre (-6.8202, -28.0261) radius 0.5
  circle A499 centre (-1.8202, -25.4742) radius 0.5
  circle A500 centre (-1.8202, -28.0262) radius 0.5
  line L221 (0, -31.6291) -> (0, -134.1173)
  line L222 (0, -26.6289) -> (0, -129.1171)
  line L223 (0, -21.6291) -> (0, -124.1173)
  line L224 (0, -16.6289) -> (0, -119.1171)
  circle A501 centre (-19.3202, -28.0001) radius 0.5
  line L225 (0, -11.6291) -> (0, -114.1173)
  line L226 (0, -11.6289) -> (0, -114.1171)
  line L227 (0, -6.6291) -> (0, -109.1173)
  line L228 (0, -6.6289) -> (0, -109.1171)
  line L229 (0, -1.6291) -> (0, -104.1173)
  line L230 (0, -1.6289) -> (0, -104.1171)
  line L231 (0, 3.3709) -> (0, -99.1173)
  line L232 (0, 3.3711) -> (0, -99.1171)
  line L233 (0, 8.3711) -> (0, -94.1171)
  circle A502 centre (-9.3202, -30.4742) radius 0.5
  circle A503 centre (-9.3202, -33.0259) radius 0.5
  circle A504 centre (-14.3202, -23.0258) radius 0.5
  circle A505 centre (-1.8202, -33.0261) radius 0.5
  circle A506 centre (-1.8202, -35.4742) radius 0.5
  circle A507 centre (-4.3202, -35.4742) radius 0.5
  circle A508 centre (-6.8202, -35.4744) radius 0.5
  circle A509 centre (-6.8202, -33.0259) radius 0.5
  circle A510 centre (-6.8202, -30.4742) radius 0.5
  line L234 (-21.5945, -25.5001) -> (0, -23.0001) construction
  line L235 (-21.5945, -23.0001) -> (0, -25.5001) construction
  circle A511 centre (-14.3202, -20.4744) radius 0.5
  circle A512 centre (-19.3202, -25.5003) radius 0.5
  circle A513 centre (-14.3202, -25.4745) radius 0.5
  circle A514 centre (-16.8202, -20.5001) radius 0.5
  circle A515 centre (-16.8202, -23) radius 0.5
  circle A516 centre (-16.8202, -25.5003) radius 0.5
  circle A517 centre (-19.3202, -23) radius 0.5
  circle A518 centre (-6.8202, -23.0259) radius 0.5
  circle A519 centre (-4.3202, -20.4741) radius 0.5
  circle A520 centre (-1.8202, -20.4741) radius 0.5
  circle A521 centre (-6.8202, -20.4742) radius 0.5
  circle A522 centre (-11.8202, -30.4744) radius 0.5
  circle A523 centre (-11.8202, -33.0258) radius 0.5
  circle A524 centre (-14.3202, -30.4744) radius 0.5
  circle A525 centre (-14.3202, -33.0258) radius 0.5
  circle A526 centre (-16.8202, -33) radius 0.5
  circle A527 centre (-16.8202, -30.5001) radius 0.5
  line L236 (0, -35.5001) -> (-21.5, -33.0001) construction
  line L237 (0, -33.0001) -> (-21.5, -35.5001) construction
  line L238 (-21.5945, -35.5001) -> (0, -33.0001) construction
  line L239 (-21.5945, -33.0001) -> (0, -35.5001) construction
  circle A528 centre (-19.3202, -33) radius 0.5
  circle A529 centre (-19.3202, -30.5001) radius 0.5
  circle A530 centre (-19.3202, -35.5003) radius 0.5
  circle A531 centre (-4.3202, -33.0261) radius 0.5
  circle A532 centre (-14.3202, -28.0259) radius 0.5
  circle A533 centre (-19.3202, -20.5001) radius 0.5
  circle A534 centre (-11.8202, -28.0259) radius 0.5
  circle A535 centre (-11.8202, -25.4745) radius 0.5
  circle A536 centre (-11.8202, -23.0258) radius 0.5
  circle A537 centre (-9.3202, -23.0259) radius 0.5
  circle A538 centre (-6.8202, -25.4744) radius 0.5
  circle A539 centre (-9.3202, -25.4744) radius 0.5
  circle A540 centre (-9.3202, -28.0261) radius 0.5
  circle A541 centre (-9.3202, -20.4742) radius 0.5
  circle A542 centre (-11.8202, -20.4744) radius 0.5
  circle A543 centre (-16.8202, -28.0001) radius 0.5
  line L240 (0, -20.5001) -> (-21.5, -18.0001) construction
  line L241 (-21.5, -18.0001) -> (0, -20.5001) construction
  line L242 (0, -18.0001) -> (-21.5, -20.5001) construction
  line L243 (-21.5, -20.5001) -> (0, -18.0001) construction
  line L244 (0, -23.0001) -> (-21.5, -25.5001) construction
  line L245 (0, -25.5001) -> (-21.5, -23.0001) construction
  line L246 (-21.5, -28.0001) -> (0, -30.5001) construction
  line L247 (-21.5, -30.5001) -> (0, -28.0001) construction
  line L248 (-21.5, -28.0001) -> (0, -30.5001) construction
  line L249 (-21.5, -30.5001) -> (0, -28.0001) construction
  line L250 (0, -111.8715) -> (0, -9.3833)
  line L251 (0, -106.8713) -> (0, -4.3832)
  line L252 (0, -96.8713) -> (0, 5.6168)
  line L253 (0, -101.8715) -> (0, 0.6167)
  line L254 (0, -91.8715) -> (0, 10.6167)
  line L255 (0, -106.8715) -> (0, -4.3833)
  line L256 (0, -71.8713) -> (0, 30.6168)
  line L257 (0, -101.8713) -> (0, 0.6168)
  line L258 (0, -96.8715) -> (0, 5.6167)
  line L259 (0, -91.8713) -> (0, 10.6168)
  line L260 (0, -86.8715) -> (0, 15.6167)
  line L261 (0, -81.8713) -> (0, 20.6168)
  line L262 (0, -76.8715) -> (0, 25.6167)
  line L263 (0, -71.8713) -> (0, 30.6168)
  line L264 (0, -51.8712) -> (0, 50.617)
  line L265 (0, -51.8713) -> (0, 50.6168)
  line L266 (0, -56.8712) -> (0, 45.617)
  line L267 (0, -56.8713) -> (0, 45.6168)
  line L268 (0, -66.8713) -> (0, 35.6168)
  line L269 (0, -66.8712) -> (0, 35.617)
  line L270 (0, -61.8712) -> (0, 40.617)
  line L271 (0, -61.8713) -> (0, 40.6168)
  line L272 (0, -36.6291) -> (0, -139.1173)
  line L273 (0, -36.6289) -> (0, -139.1171)
  line L274 (0, -31.6291) -> (0, -134.1173)
  line L275 (0, -31.6289) -> (0, -134.1171)
  line L276 (0, -26.6291) -> (0, -129.1173)
  line L277 (0, -26.6289) -> (0, -129.1171)
  line L278 (0, -21.6289) -> (0, -124.1171)
  circle A544 centre (11.8202, -35.4745) radius 0.5
  circle A545 centre (11.8202, -38.0259) radius 0.5
  line L279 (-21.7358, -35.5001) -> (21.2642, -35.5001) construction
  line L280 (-21.5945, -35.5001) -> (21.4055, -35.5001) construction
  line L281 (-20.9841, -40.5001) -> (22.0159, -40.5001) construction
  line L282 (-21.5, -36.7502) -> (21.5, -36.7502) construction
  line L283 (-21.5, -38.0001) -> (21.5, -38.0001) construction
  line L284 (-21.5, -39.2501) -> (21.5, -39.2501) construction
  line L285 (-21.5, -40.5001) -> (21.5, -40.5001) construction
  circle A546 centre (14.3202, -38.0259) radius 0.5
  circle A547 centre (6.8202, -38.0261) radius 0.5
  circle A548 centre (4.3202, -38.0262) radius 0.5
  circle A549 centre (1.8202, -38.0262) radius 0.5
  circle A550 centre (14.3202, -40.4744) radius 0.5
  circle A551 centre (11.8202, -40.4744) radius 0.5
  circle A552 centre (-4.3202, -35.4742) radius 0.5
  circle A553 centre (1.8202, -35.4742) radius 0.5
  circle A554 centre (6.8202, -35.4744) radius 0.5
  circle A555 centre (6.8202, -40.4742) radius 0.5
  circle A556 centre (4.3202, -35.4742) radius 0.5
  circle A557 centre (4.3202, -40.4741) radius 0.5
  circle A558 centre (1.8202, -40.4741) radius 0.5
  circle A559 centre (9.3202, -38.0261) radius 0.5
  circle A560 centre (9.3202, -35.4744) radius 0.5
  circle A561 centre (9.3202, -40.4742) radius 0.5
  circle A562 centre (16.8202, -40.5001) radius 0.5
  circle A563 centre (19.3202, -40.5001) radius 0.5
  circle A564 centre (14.3202, -35.4745) radius 0.5
  circle A565 centre (16.8202, -38.0001) radius 0.5
  circle A566 centre (16.8202, -35.5003) radius 0.5
  circle A567 centre (19.3202, -35.5003) radius 0.5
  circle A568 centre (19.3202, -38.0001) radius 0.5
  line L286 (0, -76.8713) -> (0, 25.6168)
  line L287 (0, -51.8713) -> (0, 50.6168)
  line L288 (0, -56.8712) -> (0, 45.617)
  line L289 (0, -56.8713) -> (0, 45.6168)
  line L290 (0, -61.8712) -> (0, 40.617)
  line L291 (0, -61.8713) -> (0, 40.6168)
  line L292 (0, -71.8713) -> (0, 30.6168)
  line L293 (0, -71.8712) -> (0, 30.617)
  line L294 (0, -66.8713) -> (0, 35.6168)
  line L295 (0, -66.8712) -> (0, 35.617)
  line L296 (0, -46.8712) -> (0, 55.617)
  line L297 (0, -41.8713) -> (0, 60.6168)
  line L298 (0, -36.8712) -> (0, 65.617)
  line L299 (0, -36.8712) -> (0, 65.617)
  circle A569 centre (-6.8202, -40.4742) radius 0.5
  circle A570 centre (-6.8202, -35.4744) radius 0.5
  circle A571 centre (-6.8202, -38.0261) radius 0.5
  circle A572 centre (-1.8202, -40.4741) radius 0.5
  circle A573 centre (-1.8202, -35.4742) radius 0.5
  circle A574 centre (-11.8202, -40.4744) radius 0.5
  circle A575 centre (-14.3202, -40.4744) radius 0.5
  circle A576 centre (-16.8202, -40.5001) radius 0.5
  circle A577 centre (-11.8202, -38.0259) radius 0.5
  circle A578 centre (-11.8202, -35.4745) radius 0.5
  circle A579 centre (-14.3202, -35.4745) radius 0.5
  circle A580 centre (-16.8202, -35.5003) radius 0.5
  circle A581 centre (-19.3202, -40.5001) radius 0.5
  circle A582 centre (-19.3202, -35.5003) radius 0.5
  circle A583 centre (-19.3202, -38.0001) radius 0.5
  circle A584 centre (-14.3202, -38.0259) radius 0.5
  circle A585 centre (-16.8202, -38.0001) radius 0.5
  line L300 (-21.5945, -35.5001) -> (0, -33.0001) construction
  line L301 (-21.5945, -33.0001) -> (0, -35.5001) construction
  line L302 (-21.5, -38.0001) -> (0, -40.5001) construction
  line L303 (-21.5, -40.5001) -> (0, -38.0001) construction
  line L304 (-21.5, -40.5001) -> (0, -38.0001) construction
  line L305 (-21.5, -38.0001) -> (0, -40.5001) construction
  line L306 (0, -35.5001) -> (-21.5, -33.0001) construction
  line L307 (0, -33.0001) -> (-21.5, -35.5001) construction
  circle A586 centre (-9.3202, -35.4744) radius 0.5
  circle A587 centre (-9.3202, -38.0261) radius 0.5
  circle A588 centre (-1.8202, -38.0262) radius 0.5
  circle A589 centre (-4.3202, -38.0262) radius 0.5
  circle A590 centre (-9.3202, -40.4742) radius 0.5
  circle A591 centre (-4.3202, -40.4741) radius 0.5
  line L308 (0, 13.3712) -> (0, -89.117)
  line L309 (0, 8.3711) -> (0, -94.1171)
  line L310 (0, 8.3712) -> (0, -94.117)
  line L311 (0, -16.6289) -> (0, -119.1171)
  line L312 (0, -11.6288) -> (0, -114.117)
  line L313 (0, -6.6289) -> (0, -109.1171)
  line L314 (0, -6.6288) -> (0, -109.117)
  line L315 (0, -1.6289) -> (0, -104.1171)
  line L316 (0, -1.6288) -> (0, -104.117)
  line L317 (0, 3.3711) -> (0, -99.1171)
  line L318 (0, 3.3712) -> (0, -99.117)
  line L319 (0, -21.6288) -> (0, -124.117)
  line L320 (0, -26.6289) -> (0, -129.1171)
  line L321 (0, -26.6289) -> (0, -129.1171)
  line L322 (0, -31.6289) -> (0, -134.1171)
  line L323 (0, -31.6291) -> (0, -134.1173)
  line L324 (0, -36.6291) -> (0, -139.1173)
  line L325 (0, -36.6289) -> (0, -139.1171)
  point P0 (0, 0)
  point P1 (3.343, 2.1853)
  point P2 (6.8797, 4.4686)
  point P3 (-13.8848, 39.5259)
  point P4 (-11.3848, 39.5259)
  point P5 (10.3145, 6.7003)
  point P6 (-13.8848, 36.9742)
  point P7 (-11.3848, 36.9742)
  point P8 (-13.8848, 31.9741)
  point P9 (-11.3848, 31.9741)
  point P10 (-11.3848, 34.5258)
  point P11 (-13.8848, 34.5258)
  point P12 (-13.8848, 21.9741)
  point P13 (-11.3848, 21.9741)
  point P14 (-11.3848, 24.5258)
  point P15 (-13.8848, 24.5258)
  point P16 (-11.3848, 29.5259)
  point P17 (-13.8848, 26.9742)
  point P18 (-13.8848, 29.5259)
  point P19 (-11.3848, 26.9742)
  point P20 (-11.3848, 19.5259)
  point P21 (-13.8848, 19.5259)
  point P22 (-13.8848, -3.0259)
  point P23 (-11.3848, -3.0259)
  point P24 (-11.3848, -0.4742)
  point P25 (-13.8848, -0.4742)
  point P26 (-11.3848, 4.5259)
  point P27 (-13.8848, 1.9742)
  point P28 (-13.8848, 4.5259)
  point P29 (-11.3848, 1.9742)
  point P30 (-11.3848, 6.9741)
  point P31 (-11.3848, 14.5259)
  point P32 (-13.8848, 14.5259)
  point P33 (-13.8848, 11.9742)
  point P34 (-13.8848, 6.9741)
  point P35 (-11.3848, 9.5258)
  point P36 (-11.3848, 11.9742)
  point P37 (-13.8848, 9.5258)
  point P38 (-11.3848, 16.9741)
  point P39 (-13.8848, 16.9741)
  point P40 (0, -3.5001)
  point P41 (3.343, -5.6854)
  point P42 (6.8797, -7.9687)
  point P43 (10.3145, -10.2004)
  point P44 (-13.8848, -15.4744)
  point P45 (-13.8848, -10.4742)
  point P46 (-13.8848, -8.0261)
  point P47 (-11.3848, -8.0261)
  point P48 (-11.3848, -18.0261)
  point P49 (-13.8848, -18.0261)
  point P50 (-11.3848, -3.0259)
  point P51 (-13.8848, -3.0259)
  point P52 (-13.8848, -5.4744)
  point P53 (-11.3848, -5.4744)
  point P54 (-11.3848, -10.4742)
  point P55 (-11.3848, -13.0259)
  point P56 (-11.3848, -20.4742)
  point P57 (-13.8848, -20.4742)
  point P58 (-13.8848, -13.0259)
  point P59 (-11.3848, -15.4744)
  point P60 (-13.8848, -35.4744)
  point P61 (-11.3848, -35.4744)
  point P62 (0, -35.0001)
  point P63 (10.3145, -28.2999)
  point P64 (3.343, -32.8149)
  point P65 (6.8797, -30.5316)
  point P66 (-13.8848, -20.4742)
  point P67 (-11.3848, -30.4742)
  point P68 (-11.3848, -20.4742)
  point P69 (-11.3848, -33.0259)
  point P70 (-13.8848, -23.0259)
  point P71 (-13.8848, -28.0261)
  point P72 (-13.8848, -30.4742)
  point P73 (-13.8848, -33.0259)
  point P74 (-13.8848, -35.4744)
  point P75 (-11.3848, -35.4744)
  point P76 (-11.3848, -28.0261)
  point P77 (-11.3848, -25.4744)
  point P78 (-11.3848, -23.0259)
  point P79 (-13.8848, -25.4744)
  point P80 (10.3145, -40.2004)
  point P81 (6.8797, -37.9687)
  point P82 (3.343, -35.6854)
  point P83 (-11.3848, -40.4742)
  point P84 (-13.8848, -40.4742)